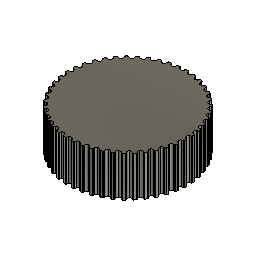
gear_47z (Autodesk Fusion 360 design; units mm, degrees)
Autodesk Fusion 360 part; units mm, degrees
sketch "Sketch1" plane through (0, 0, 0) normal (0, 0, 1) x (1, 0, 0) in component "gt2 pulley"
  circle A0 centre (0, 0) radius 14.9606 construction
  circle A1 centre (0, 0) radius 13.9566 construction
  line L0 (0, 0) -> (0, 14.9606) construction
  line L1 (0, 0) -> (0.9993, 14.9272) construction
  line L2 (0, 0) -> (1.4076, 14.8942) construction
  circle A2 centre (0, 0) radius 14.7066 construction
  arc A3 (0.3865, 14.5659) -> (0.4524, 14.2769) centre (1.3837, 14.6413) ccw
  circle A4 centre (0, 0) radius 14.5566 construction
  arc A5 (0.2393, 14.7046) -> (0, 14.7066) centre (0, 0) ccw
  arc A6 (0.3865, 14.5659) -> (0.2393, 14.7046) centre (0.2369, 14.5546) ccw
  arc A7 (0.4524, 14.2769) -> (0.9322, 13.9254) centre (0.9693, 14.4792) ccw
  arc A8 (0, 14.7066) -> (-0.2393, 14.7046) centre (0, 0) ccw
  arc A9 (-0.2393, 14.7046) -> (-0.3865, 14.5659) centre (-0.2369, 14.5546) ccw
  arc A10 (-0.4524, 14.2769) -> (-0.3865, 14.5659) centre (-1.3837, 14.6413) ccw
  arc A11 (-0.9322, 13.9254) -> (-0.4524, 14.2769) centre (-0.9693, 14.4792) ccw
  arc A12 (0.9322, 13.9254) -> (-0.9322, 13.9254) centre (0, 0) ccw
  point P0 (1.3837, 14.6413)
  point P1 (0, 14.7066)
  dimension "d18" = 29.9211
  dimension "d19" = 3.83
  dimension "d22" = 1.004
  dimension "d24" = 0.75
  dimension "d26" = 1
  dimension "d27" = 0.15
  dimension "d28" = 0.15
  dimension "d47" = 0.555
  dimension "d52" = 3.812
  constraint coincident A0.centre A1.centre
  constraint coincident A0 L0.end
  constraint vertical L0
  constraint coincident A0 L1.end
  constraint coincident A0 L2.end
  constraint concentric A1 A2
  constraint coincident A1 A7.end
  constraint coincident L1 A7.end
  constraint coincident A2 P0
  constraint coincident L2 P0
  constraint coincident P0 A3.centre
  constraint coincident A2 P1
  constraint coincident L0 P1
  constraint concentric A2 A4
  constraint coincident P1 A5.end
  constraint coincident A4 A6.centre
  constraint coincident A3.start A6.start
  constraint tangent A3 A6
  constraint tangent A3 A7
  constraint symmetric L0 A7.end A11.start
  constraint symmetric L0 A3.start A9.end
  constraint symmetric L0 A3.end A10.start
  constraint symmetric L0 A3 A10
  constraint symmetric L0 A5.start A8.end
  constraint symmetric L0 P1 A5.end
  constraint symmetric L0 A5 A8
  constraint symmetric L0 A6 A9
  constraint symmetric L0 A7 A11
  constraint coincident A1 A11.start
  constraint tangent A1 A7
  constraint coincident L1 A7.centre
  measures "d18" diameter of A0
  measures "d19" angle of L0 L1
  measures "d22" distance of A0 A1
  measures "d24" distance of A1 A2
  measures "d26" radius of A3
  measures "d27" distance of A2 A4
  measures "d28" radius of A6
  measures "d47" radius of A7
extrude "Extrude1" add sketch "Sketch1" along normal blind 10 makes body 1
pattern_circular "C-Pattern1" count 47 over 360 about axis through (0, 0, 1.75) along (0, 0, 1) of bodies 1 makes body 2 at (-1.9629, 13.8178, 6.6667) makes body 3 at (-3.7871, 13.4329, 6.6667) makes body 4 at (-5.5438, 12.8083, 6.6667) makes body 5 at (-7.7269, 11.6224, 6.6667) makes body 6 at (-8.7307, 10.8886, 6.6667) makes body 7 at (-10.5229, 9.1681, 6.6667) makes body 8 at (-10.7906, 8.8514, 3.3333) makes body 9 at (-12.2887, 6.6162, 6.6667) makes body 10 at (-12.7457, 5.6861, 3.3333) makes body 11 at (-13.6, 3.1345, 6.6667) makes body 12 at (-13.8965, 1.2938, 6.6667) makes body 13 at (-13.9542, 0.2591, 3.3333) makes body 14 at (-13.6229, -3.0334, 6.6667) makes body 15 at (-13.5268, -3.4367, 3.3333) makes body 16 at (-12.6159, -5.9687, 6.6667) makes body 17 at (-12.1382, -6.8883, 3.3333) makes body 18 at (-10.1753, -9.5524, 6.6667) makes body 19 at (-8.8113, -10.8234, 6.6667) makes body 20 at (-8.4859, -11.0804, 3.3333) makes body 21 at (-5.6387, -12.7668, 6.6667) makes body 22 at (-4.4801, -13.218, 6.6667) makes body 23 at (-2.6783, -13.6972, 6.6667) makes body 24 at (-1.6546, -13.8581, 3.3333) makes body 25 at (1.0356, -13.9181, 6.6667) makes body 26 at (2.8815, -13.6559, 6.6667) makes body 27 at (3.8868, -13.4044, 3.3333) makes body 28 at (6.9334, -12.1126, 6.6667) makes body 29 at (7.9839, -11.4474, 6.6667) makes body 30 at (9.4385, -10.2811, 6.6667) makes body 31 at (11.1118, -8.4447, 6.6667) makes body 32 at (12.1382, -6.8883, 6.6667) makes body 33 at (12.3375, -6.5247, 3.3333) makes body 34 at (13.5268, -3.4367, 6.6667) makes body 35 at (13.8642, -1.6031, 6.6667) makes body 36 at (13.9518, -0.3627, 6.6667) makes body 37 at (13.8757, 1.5001, 6.6667) makes body 38 at (13.552, 3.3362, 6.6667) makes body 39 at (12.7457, 5.6861, 6.6667) makes body 40 at (11.8741, 7.3342, 6.6667) makes body 41 at (10.7906, 8.8514, 6.6667) makes body 42 at (10.5229, 9.1681, 3.3333) makes body 43 at (8.568, 11.017, 6.6667) makes body 44 at (7.7269, 11.6224, 3.3333) makes body 45 at (6.1088, 12.5486, 3.3333) makes body 46 at (4.3818, 13.2509, 3.3333) makes body 47 at (2.5765, 13.7167, 3.3333)
sketch "Sketch2" plane through (0, 0, 10) normal (0, 0, 1) x (-1, 0, 0)
  arc A0 (-9.3306, -11.1918) -> (-9.301, -11.3919) centre (-9.2062, -11.2756) ccw
  arc A1 (-9.301, -11.3919) -> (-8.9254, -11.6885) centre (0, 0) ccw
  arc A2 (-8.9254, -11.6885) -> (-8.7239, -11.6709) centre (-8.8343, -11.5693) ccw
  arc A3 (-8.493, -11.4849) -> (-8.7239, -11.6709) centre (-7.9881, -12.348) ccw
  arc A4 (-7.8987, -11.5064) -> (-8.493, -11.4849) centre (-8.2128, -11.9639) ccw
  arc A5 (-9.3619, -10.3509) -> (-7.8987, -11.5064) centre (0, 0) ccw
  arc A6 (-9.2032, -10.9241) -> (-9.3619, -10.3509) centre (-9.7341, -10.7625) ccw
  arc A7 (-9.3306, -11.1918) -> (-9.2032, -10.9241) centre (-10.1599, -10.633) ccw
  circle A8 centre (0, 0) radius 13.9566
  constraint concentric A1 A8
extrude "Extrude2" add sketch "Sketch2" against normal blind 10 contours A5 A8 bodies 1 2 3 4 5 6 7 8 9 10 11 12 13 14 15 16 17 18 19 20 21 22 23 24 25 26 27 28 29 30 31 32 33 34 35 36 37 38 39 40 41 42 43 44 45 46 47
extrude "Extrude4" [suppressed] in component "gt2 pulley"
pattern_circular "C-Pattern7" [suppressed] in component "gt2 pulley"
extrude "Extrude3" [suppressed] in component "gt2 pulley"
pattern_circular "C-Pattern6" [suppressed] in component "gt2 pulley"
extrude "Extrude2'" [suppressed] in component "gt2 pulley"
pattern_circular "C-Pattern5" [suppressed] in component "gt2 pulley"
extrude "Extrude1'" [suppressed] in component "gt2 pulley"
pattern_circular "C-Pattern4" [suppressed] in component "gt2 pulley"
pattern_circular "C-Pattern3" [suppressed] in component "gt2 pulley"
pattern_circular "C-Pattern2" [suppressed] in component "gt2 pulley"
pattern_circular "C-Pattern1'" [suppressed] in component "gt2 pulley"
copy_body "Body->Comp1" [suppressed] in component "Component"
copy_body "Body->Comp2" [suppressed] in component "Component'"
copy_body "Body->Comp3" [suppressed] in component "Component''"
copy_body "Body->Comp4" [suppressed] in component "Component'''"
copy_body "Body->Comp5" [suppressed] in component "Component''''"
copy_body "Body->Comp6" [suppressed] in component "Component'''''"
copy_body "Body->Comp7" [suppressed] in component "Component''''''"
copy_body "Body->Comp8" [suppressed] in component "Component'''''''"
copy_body "Body->Comp9" [suppressed] in component "Component''''''''"
copy_body "Body->Comp10" [suppressed] in component "Component'''''''''"
copy_body "Body->Comp11" [suppressed] in component "Component''''''''''"
copy_body "Body->Comp12" [suppressed] in component "Component'''''''''''"
copy_body "Body->Comp13" [suppressed] in component "Component''''''''''''"
copy_body "Body->Comp14" [suppressed] in component "Component'''''''''''''"
copy_body "Body->Comp15" [suppressed] in component "Component''''''''''''''"
copy_body "Body->Comp16" [suppressed] in component "Component'''''''''''''''"
copy_body "Body->Comp17" [suppressed] in component "Component''''''''''''''''"
copy_body "Body->Comp18" [suppressed] in component "Component'''''''''''''''''"
copy_body "Body->Comp19" [suppressed] in component "Component''''''''''''''''''"
copy_body "Body->Comp20" [suppressed] in component "Component'''''''''''''''''''"
component "gt2 pulley" placed x (1, 0, 0) y (0, 1, 0) z (0, 0, 1) at (0, 0, 0)
equation "NumTeeth = 47" comment "min 20"
equation "ToothPitch = 2 mm"
equation "PullyDia = NumTeeth * ToothPitch / PI"
equation "ToothAng = ( ( 360 / NumTeeth ) * 1 deg )"
equation "TransOffsetAngle = ToothAng * 0.2"
equation "Sholulder_Radius = 0.15 mm"
equation "Root_Radius = 0.555 mm"
equation "TransRadius = 1 mm"
equation "ToolHeight = 0.75 mm"
equation "PLD = 0.254 mm"
equation "d18 = PullyDia"
equation "d19 = ToothAng / 2"
equation "d22 = PLD + ToolHeight"
equation "d24 = ToolHeight"
equation "d26 = TransRadius"
equation "d27 = Sholulder_Radius"
equation "d31 = NumTeeth"
equation "d33 = NumTeeth"
equation "d35 = NumTeeth"
equation "d37 = NumTeeth"
equation "d41 = NumTeeth"
equation "d45 = NumTeeth"
equation "d47 = Root_Radius"
equation "d50 = NumTeeth"
